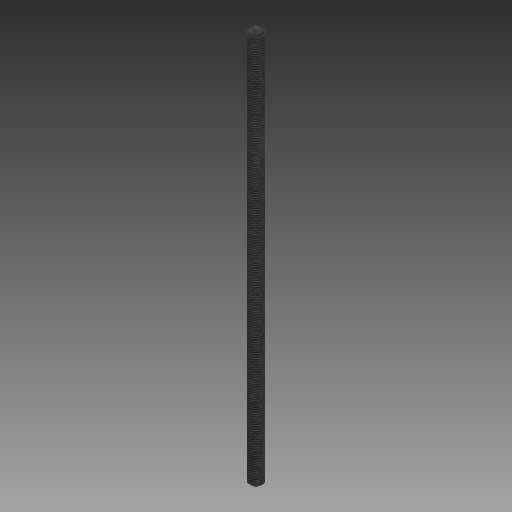
# Autodesk Inventor part: Gewindestange M3x91mm
Saved by Autodesk Inventor 2018 (Build 220112000, 112)
## iProperties
Created: 2019-03-04
Part Number: Gewindestange M3x91mm
Material: Stahl
Document SubType Name: Modeling
Designer: RedBots
Density: 7.85 g/cm^3
Appearance: Platte
Mass: 5.04323 g
Surface Area: 8.68245 cm^2
Volume: 0.642449 cm^3
Author: RedBots
Autodesk Inventor part; units mm, degrees
ref_plane "YZ Plane" through (0, 0, 0) normal (1, 0, 0) x (0, 1, 0)
ref_plane "XZ Plane" through (0, 0, 0) normal (0, 1, 0) x (-1, 0, 0)
ref_plane "XY Plane" through (0, 0, 0) normal (0, 0, 1) x (1, 0, 0)
sketch "Skizze1" plane through (0, 0, 0) normal (0, 0, 1) x (1, 0, 0)
  circle A0 centre (0, 0) radius 1.5
  dimension "d0" = 3
  constraints: 1 centre point, 1 coincident
  measures "d0" diameter of A0
extrude "Extrusion1" add sketch "Skizze1" along normal blind 91
thread "Gewinde1" size "M3x0.5" class "6g" standard "ANSI Metric M Profile" full length
chamfer "Fase1" distance 0.3 angle 45 2 edges at (-1.5, 0, 91) (-1.5, 0, 0)
